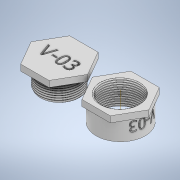
# Autodesk Inventor part: boltAndNut1_625x12-V03
Saved by Autodesk Inventor 2021.1 (Build 251245000, 245)
## iProperties
Created: 2020-08-22
Part Number: boltAndNut1_625x12-V03
Material: Generic
Document SubType Name: Modeling
Designer: robst
Density: 1 g/cm^3
Appearance: Default
Author: robst
Autodesk Inventor part; units mm, degrees
ref_plane "XZ Plane" through (0, 0, 0) normal (0, 1, 0) x (-1, 0, 0)
ref_plane "XY Plane" through (0, 0, 0) normal (0, 0, 1) x (1, 0, 0)
sketch "Sketch4" plane through (0, 0, 0) normal (0, 1, 0) x (-1, 0, 0)
  circle A0 centre (0, 0) radius 25.4
  circle A1 centre (0, 0) radius 19.7206
  dimension "d4" = 50.8
  dimension "d5" = 39.4411
  constraints: 2 centre point, 2 coincident
  measures "d4" diameter of A0
  measures "d5" diameter of A1
extrude "NutShaft" add sketch "Sketch4" against normal blind 25.4
sketch "Sketch6" plane through (0, 0, 0) normal (0, 0, 1) x (1, 0, 0)
  line L0 (19.7206, -25.4) -> (19.7206, 0) projected
  line L1 (19.7206, 2.1167) -> (20.8305, 2.7575)
  line L2 (20.8305, 2.9555) -> (19.7206, 3.5963)
  line L3 (19.7206, 3.5963) -> (19.7206, 2.1167)
  line L4 (0, -31.1993) -> (0, 9.3956) projected
  arc A0 (20.8305, 2.7575) -> (20.8305, 2.9555) centre (20.7734, 2.8565) ccw
  point P0 (0, 0)
  dimension "d33" = 60
  dimension "d35" = 0.1143
  dimension "d36" = 20.8877
  dimension "d37" = 2.1167
  dimension "d78" = 19.7206
  constraints: 6 end point, 2 point on circle, 2 tangent, 1 centre point, 1 collinear, 1 equal length, 1 vertical
  measures "d33" angle of L1 L2
  measures "d35" radius of A0
  measures "d37" distance of L1.start L0.end
  measures "d78" distance between parallel lines of L3 L4
coil "CoilForNut" sketch "Sketch6" operation cut axis through (0, -10, 0) along (0, -1, 0) pitch 2.1167 turns 14 hand right
sketch "Sketch7" plane through (0, 0, 0) normal (0, 1, 0) x (-1, 0, 0)
  line L0 (0, 0) -> (63.5, 0) construction
  line L1 (34.1706, 0) -> (48.8353, 25.4)
  line L2 (48.8353, 25.4) -> (78.1647, 25.4)
  line L3 (78.1647, 25.4) -> (92.8294, 0)
  line L4 (92.8294, 0) -> (78.1647, -25.4)
  line L5 (78.1647, -25.4) -> (48.8353, -25.4)
  line L6 (48.8353, -25.4) -> (34.1706, 0)
  dimension "d46" = 63.5
  dimension "d50" = 50.8
  constraints: 14 end point, 2 horizontal, 1 coincident, 13 other
  measures "d46" distance of L0.start L0.end
  measures "d50" distance between parallel lines of L2 L5
extrude "BoltHexHead" add sketch "Sketch7" against normal blind 6.35
sketch "Sketch8" plane through (0, -6.35, 0) normal (0, -1, 0) x (1, 0, 0)
  line L0 (-48.8353, 25.4) -> (-78.1647, 25.4) projected
  line L1 (-34.1706, 0) -> (-48.8353, 25.4) projected
  line L2 (-48.8353, -25.4) -> (-34.1706, 0) projected
  line L3 (-78.1647, -25.4) -> (-48.8353, -25.4) projected
  line L4 (-92.8294, 0) -> (-78.1647, -25.4) projected
  line L5 (-78.1647, 25.4) -> (-92.8294, 0) projected
  line L6 (-78.1647, 25.4) -> (-69.0759, -25.4) construction
  line L7 (-48.8353, 25.4) -> (-78.1647, -25.4) construction
  circle A0 centre (-63.5, 0) radius 20.4699
  point P0 (0, 0)
  dimension "d49" = 40.9397
  constraints: 4 end point, 1 centre point, 1 midpoint, 1 parallel, 1 point on line
  measures "d49" diameter of A0
extrude "BoltShaft" add sketch "Sketch8" along normal blind 19.05 contours A0
sketch "Sketch9" plane through (0, 0, 0) normal (0, 0, 1) x (1, 0, 0)
  line L0 (-43.0301, -6.35) -> (-43.0301, -25.4) projected
  line L1 (-83.9699, -25.4) -> (-43.0301, -25.4) projected
  line L2 (-43.0301, -27.5167) -> (-44.3116, -28.2565)
  line L3 (-44.3116, -28.5821) -> (-43.0301, -29.3219)
  line L4 (-43.0301, -29.3219) -> (-43.0301, -27.5167)
  line L5 (-63.5, -25.4) -> (-63.5, 0) construction
  line L6 (-78.1647, 0) -> (-48.8353, 0) construction
  arc A0 (-44.3116, -28.2565) -> (-44.3116, -28.5821) centre (-44.2176, -28.4193) ccw
  point P0 (0, 0)
  dimension "d53" = 60
  dimension "d54" = 0.188
  dimension "d56" = 20.4699
  dimension "d57" = 19.0944
  dimension "d66" = 2.1167
  constraints: 8 end point, 2 midpoint, 2 point on circle, 2 tangent, 1 centre point, 1 equal length
  measures "d53" angle of L2 L3
  measures "d54" radius of A0
  measures "d56" distance between parallel lines of L4 L5
  measures "d57" distance edge to line of A0 L5
  measures "d66" distance of L2.start L0.end
coil "CoilForBolt" sketch "Sketch9" operation cut axis through (-63.5, -25.4, 0) along (0, 1, 0) pitch 2.1167 turns 10 hand right
sketch "Sketch11" plane through (0, 0, 0) normal (0, 1, 0) x (1, 0, 0)
  line L0 (-78.1647, -25.4) -> (-92.8294, 0) construction
  line L1 (-48.8353, 25.4) -> (-34.1706, 0) construction
  line L2 (-92.8294, 0) -> (-34.1706, 0) construction
  line L3 (-70.9152, 6.35) -> (-75.2892, -6.35)
  line L4 (-75.2892, -6.35) -> (-77.1108, -6.35)
  line L5 (-77.1108, -6.35) -> (-81.4848, 6.35)
  line L6 (-81.4848, 6.35) -> (-79.6735, 6.35)
  line L7 (-79.6735, 6.35) -> (-76.1537, -4.199)
  line L8 (-76.1537, -4.199) -> (-72.6339, 6.35)
  line L9 (-72.6339, 6.35) -> (-70.9152, 6.35)
  line L10 (-65.265, -1.5643) -> (-70.0713, -1.5643)
  line L11 (-70.0713, -1.5643) -> (-70.0713, -0.0206)
  line L12 (-70.0713, -0.0206) -> (-65.265, -0.0206)
  line L13 (-65.265, -0.0206) -> (-65.265, -1.5643)
  spline S0 degree 2 poles (-55.6731, 0) (-55.6731, -3.4169) (-57.6594, -6.6176) (-59.7281, -6.6176) knots 0 0 0 1 2 2 2
  spline S1 degree 2 poles (-59.7281, -6.6176) (-61.8276, -6.6176) (-63.7933, -3.3551) (-63.7933, -0.0103) knots 0 0 0 1 2 2 2
  spline S2 degree 2 poles (-63.7933, -0.0103) (-63.7933, 3.4271) (-61.807, 6.6073) (-59.7281, 6.6073) knots 0 0 0 1 2 2 2
  spline S3 degree 2 poles (-59.7281, 6.6073) (-57.6389, 6.6073) (-55.6731, 3.3139) (-55.6731, 0) knots 0 0 0 1 2 2 2
  spline S4 degree 2 poles (-57.855, -3.8697) (-57.608, -3.2419) (-57.4021, -1.3071) (-57.4021, 0) knots 0 0 0 1 2 2 2
  spline S5 degree 2 poles (-57.4021, 0) (-57.4021, 1.3071) (-57.608, 3.2316) (-57.8653, 3.88) knots 0 0 0 1 2 2 2
  spline S6 degree 2 poles (-57.8653, 3.88) (-58.1226, 4.5284) (-59.0179, 5.1973) (-59.7281, 5.1973) knots 0 0 0 1 2 2 2
  spline S7 degree 2 poles (-59.7281, 5.1973) (-60.4382, 5.1973) (-61.3542, 4.5284) (-61.6218, 3.8594) knots 0 0 0 1 2 2 2
  spline S8 degree 2 poles (-61.6218, 3.8594) (-61.8791, 3.211) (-62.0643, 1.235) (-62.0643, -0.0103) knots 0 0 0 1 2 2 2
  spline S9 degree 2 poles (-62.0643, -0.0103) (-62.0643, -1.3482) (-61.8996, -3.139) (-61.632, -3.8388) knots 0 0 0 1 2 2 2
  spline S10 degree 2 poles (-61.632, -3.8388) (-61.385, -4.4975) (-60.4691, -5.2076) (-59.7281, -5.2076) knots 0 0 0 1 2 2 2
  spline S11 degree 2 poles (-59.7281, -5.2076) (-59.0282, -5.2076) (-58.1123, -4.5387) (-57.855, -3.8697) knots 0 0 0 1 2 2 2
  spline S12 degree 2 poles (-50.6199, 5.1459) (-51.083, 5.1459) (-51.999, 4.9194) (-52.4415, 4.7445) knots 0 0 0 1 2 2 2
  spline S13 degree 2 poles (-52.4415, 4.7445) (-52.8532, 4.5695) (-53.4604, 4.199) (-53.6971, 4.0344) knots 0 0 0 1 2 2 2
  line L14 (-53.6971, 4.0344) -> (-53.8, 4.0344)
  line L15 (-53.8, 4.0344) -> (-53.8, 5.8354)
  spline S14 degree 2 poles (-53.8, 5.8354) (-53.2443, 6.1339) (-51.3403, 6.6176) (-50.4861, 6.6176) knots 0 0 0 1 2 2 2
  spline S15 degree 2 poles (-50.4861, 6.6176) (-49.6216, 6.6176) (-48.3351, 6.2677) (-47.8103, 5.8972) knots 0 0 0 1 2 2 2
  spline S16 degree 2 poles (-47.8103, 5.8972) (-47.2545, 5.4958) (-46.6782, 4.3328) (-46.6782, 3.5506) knots 0 0 0 1 2 2 2
  spline S17 degree 2 poles (-46.6782, 3.5506) (-46.6782, 2.5009) (-48.0573, 0.916) (-49.0247, 0.7101) knots 0 0 0 1 2 2 2
  line L16 (-49.0247, 0.7101) -> (-49.0247, 0.5866)
  spline S18 degree 2 poles (-49.0247, 0.5866) (-48.6233, 0.5043) (-47.7073, 0.1338) (-47.3162, -0.2367) knots 0 0 0 1 2 2 2
  spline S19 degree 2 poles (-47.3162, -0.2367) (-46.9252, -0.5969) (-46.4312, -1.7496) (-46.4312, -2.5832) knots 0 0 0 1 2 2 2
  spline S20 degree 2 poles (-46.4312, -2.5832) (-46.4312, -3.4374) (-47.0178, -4.8886) (-47.553, -5.4443) knots 0 0 0 1 2 2 2
  spline S21 degree 2 poles (-47.553, -5.4443) (-48.1087, -6.0207) (-49.6833, -6.6176) (-50.6816, -6.6176) knots 0 0 0 1 2 2 2
  spline S22 degree 2 poles (-50.6816, -6.6176) (-51.6388, -6.6176) (-53.5119, -6.1545) (-54.15, -5.8354) knots 0 0 0 1 2 2 2
  line L17 (-54.15, -5.8354) -> (-54.15, -4.0344)
  line L18 (-54.15, -4.0344) -> (-54.0265, -4.0344)
  spline S23 degree 2 poles (-54.0265, -4.0344) (-53.4913, -4.4254) (-51.6799, -5.1459) (-50.7846, -5.1459) knots 0 0 0 1 2 2 2
  spline S24 degree 2 poles (-50.7846, -5.1459) (-50.2597, -5.1459) (-49.2099, -4.8165) (-48.86, -4.4357) knots 0 0 0 1 2 2 2
  spline S25 degree 2 poles (-48.86, -4.4357) (-48.5204, -4.0549) (-48.1602, -3.1493) (-48.1602, -2.4597) knots 0 0 0 1 2 2 2
  spline S26 degree 2 poles (-48.1602, -2.4597) (-48.1602, -1.7702) (-48.5615, -0.8748) (-48.9218, -0.6175) knots 0 0 0 1 2 2 2
  spline S27 degree 2 poles (-48.9218, -0.6175) (-49.282, -0.3602) (-50.2597, -0.1647) (-50.836, -0.1647) knots 0 0 0 1 2 2 2
  line L19 (-50.836, -0.1647) -> (-51.5564, -0.1647)
  line L20 (-51.5564, -0.1647) -> (-51.5564, 1.2453)
  line L21 (-51.5564, 1.2453) -> (-50.9904, 1.2453)
  spline S28 degree 2 poles (-50.9904, 1.2453) (-49.848, 1.2453) (-48.4072, 2.3362) (-48.4072, 3.3757) knots 0 0 0 1 2 2 2
  spline S29 degree 2 poles (-48.4072, 3.3757) (-48.4072, 3.8594) (-48.7777, 4.5489) (-49.0761, 4.7548) knots 0 0 0 1 2 2 2
  spline S30 degree 2 poles (-49.0761, 4.7548) (-49.3952, 4.9709) (-50.1774, 5.1459) (-50.6199, 5.1459) knots 0 0 0 1 2 2 2
  point P0 (0, 0)
  constraints: 2 end point, 2 horizontal
extrude "EmbossForBolt" cut sketch "Sketch11" against normal blind 2.54
ref_plane "Work Plane4" through (25.4, 0, 0) normal (1, 0, 0) x (0, 1, 0)
sketch "Sketch12" plane through (25.4, 0, 0) normal (1, 0, 0) x (0, 1, 0)
  line L0 (0, 25.4) -> (-25.4, 25.4)
  line L1 (0, -25.4) -> (0, 25.4)
  line L2 (0, -25.4) -> (-25.4, -25.4)
  line L3 (-25.4, 25.4) -> (-25.4, -25.4) projected
  line L4 (-12.7, 25.4) -> (-12.7, -25.4) construction
  line L5 (-17.78, -5.9322) -> (-7.62, -9.4313)
  line L6 (-7.62, -9.4313) -> (-7.62, -10.8887)
  line L7 (-7.62, -10.8887) -> (-17.78, -14.3878)
  line L8 (-17.78, -14.3878) -> (-17.78, -12.9388)
  line L9 (-17.78, -12.9388) -> (-9.3408, -10.1229)
  line L10 (-9.3408, -10.1229) -> (-17.78, -7.3071)
  line L11 (-17.78, -7.3071) -> (-17.78, -5.9322)
  line L12 (-11.4485, -1.412) -> (-11.4485, -5.257)
  line L13 (-11.4485, -5.257) -> (-12.6835, -5.257)
  line L14 (-12.6835, -5.257) -> (-12.6835, -1.412)
  line L15 (-12.6835, -1.412) -> (-11.4485, -1.412)
  spline S0 degree 2 poles (-12.7, 6.2615) (-9.9665, 6.2615) (-7.4059, 4.6724) (-7.4059, 3.0175) knots 0 0 0 1 2 2 2
  spline S1 degree 2 poles (-7.4059, 3.0175) (-7.4059, 1.3379) (-10.0159, -0.2347) (-12.6918, -0.2347) knots 0 0 0 1 2 2 2
  spline S2 degree 2 poles (-12.6918, -0.2347) (-15.4417, -0.2347) (-17.9858, 1.3544) (-17.9858, 3.0175) knots 0 0 0 1 2 2 2
  spline S3 degree 2 poles (-17.9858, 3.0175) (-17.9858, 4.6889) (-15.3512, 6.2615) (-12.7, 6.2615) knots 0 0 0 1 2 2 2
  spline S4 degree 2 poles (-9.6042, 4.516) (-10.1065, 4.7136) (-11.6544, 4.8783) (-12.7, 4.8783) knots 0 0 0 1 2 2 2
  spline S5 degree 2 poles (-12.7, 4.8783) (-13.7456, 4.8783) (-15.2853, 4.7136) (-15.804, 4.5078) knots 0 0 0 1 2 2 2
  spline S6 degree 2 poles (-15.804, 4.5078) (-16.3227, 4.3019) (-16.8579, 3.5856) (-16.8579, 3.0175) knots 0 0 0 1 2 2 2
  spline S7 degree 2 poles (-16.8579, 3.0175) (-16.8579, 2.4494) (-16.3227, 1.7167) (-15.7875, 1.5026) knots 0 0 0 1 2 2 2
  spline S8 degree 2 poles (-15.7875, 1.5026) (-15.2688, 1.2968) (-13.688, 1.1486) (-12.6918, 1.1486) knots 0 0 0 1 2 2 2
  spline S9 degree 2 poles (-12.6918, 1.1486) (-11.6214, 1.1486) (-10.1888, 1.2803) (-9.6289, 1.4944) knots 0 0 0 1 2 2 2
  spline S10 degree 2 poles (-9.6289, 1.4944) (-9.102, 1.692) (-8.5339, 2.4247) (-8.5339, 3.0175) knots 0 0 0 1 2 2 2
  spline S11 degree 2 poles (-8.5339, 3.0175) (-8.5339, 3.5774) (-9.0691, 4.3102) (-9.6042, 4.516) knots 0 0 0 1 2 2 2
  spline S12 degree 2 poles (-16.8167, 10.3041) (-16.8167, 9.9336) (-16.6356, 9.2008) (-16.4956, 8.8468) knots 0 0 0 1 2 2 2
  spline S13 degree 2 poles (-16.4956, 8.8468) (-16.3556, 8.5174) (-16.0592, 8.0317) (-15.9275, 7.8423) knots 0 0 0 1 2 2 2
  line L16 (-15.9275, 7.8423) -> (-15.9275, 7.76)
  line L17 (-15.9275, 7.76) -> (-17.3683, 7.76)
  spline S14 degree 2 poles (-17.3683, 7.76) (-17.6071, 8.2046) (-17.9941, 9.7277) (-17.9941, 10.4111) knots 0 0 0 1 2 2 2
  spline S15 degree 2 poles (-17.9941, 10.4111) (-17.9941, 11.1027) (-17.7141, 12.1319) (-17.4177, 12.5518) knots 0 0 0 1 2 2 2
  spline S16 degree 2 poles (-17.4177, 12.5518) (-17.0966, 12.9964) (-16.1663, 13.4575) (-15.5405, 13.4575) knots 0 0 0 1 2 2 2
  spline S17 degree 2 poles (-15.5405, 13.4575) (-14.7007, 13.4575) (-13.4328, 12.3542) (-13.2681, 11.5803) knots 0 0 0 1 2 2 2
  line L18 (-13.2681, 11.5803) -> (-13.1693, 11.5803)
  spline S18 degree 2 poles (-13.1693, 11.5803) (-13.1034, 11.9014) (-12.807, 12.6341) (-12.5106, 12.947) knots 0 0 0 1 2 2 2
  spline S19 degree 2 poles (-12.5106, 12.947) (-12.2225, 13.2599) (-11.3003, 13.6551) (-10.6334, 13.6551) knots 0 0 0 1 2 2 2
  spline S20 degree 2 poles (-10.6334, 13.6551) (-9.95, 13.6551) (-8.7891, 13.1858) (-8.3445, 12.7576) knots 0 0 0 1 2 2 2
  spline S21 degree 2 poles (-8.3445, 12.7576) (-7.8835, 12.313) (-7.4059, 11.0533) (-7.4059, 10.2547) knots 0 0 0 1 2 2 2
  spline S22 degree 2 poles (-7.4059, 10.2547) (-7.4059, 9.489) (-7.7764, 7.9905) (-8.0317, 7.48) knots 0 0 0 1 2 2 2
  line L19 (-8.0317, 7.48) -> (-9.4725, 7.48)
  line L20 (-9.4725, 7.48) -> (-9.4725, 7.5788)
  spline S23 degree 2 poles (-9.4725, 7.5788) (-9.1596, 8.007) (-8.5833, 9.456) (-8.5833, 10.1724) knots 0 0 0 1 2 2 2
  spline S24 degree 2 poles (-8.5833, 10.1724) (-8.5833, 10.5923) (-8.8468, 11.4321) (-9.1514, 11.712) knots 0 0 0 1 2 2 2
  spline S25 degree 2 poles (-9.1514, 11.712) (-9.456, 11.9837) (-10.1806, 12.2719) (-10.7322, 12.2719) knots 0 0 0 1 2 2 2
  spline S26 degree 2 poles (-10.7322, 12.2719) (-11.2839, 12.2719) (-12.0002, 11.9508) (-12.206, 11.6626) knots 0 0 0 1 2 2 2
  spline S27 degree 2 poles (-12.206, 11.6626) (-12.4118, 11.3744) (-12.5683, 10.5923) (-12.5683, 10.1312) knots 0 0 0 1 2 2 2
  line L21 (-12.5683, 10.1312) -> (-12.5683, 9.5548)
  line L22 (-12.5683, 9.5548) -> (-13.6962, 9.5548)
  line L23 (-13.6962, 9.5548) -> (-13.6962, 10.0077)
  spline S28 degree 2 poles (-13.6962, 10.0077) (-13.6962, 10.9216) (-14.569, 12.0743) (-15.4006, 12.0743) knots 0 0 0 1 2 2 2
  spline S29 degree 2 poles (-15.4006, 12.0743) (-15.7875, 12.0743) (-16.3392, 11.7779) (-16.5038, 11.5391) knots 0 0 0 1 2 2 2
  spline S30 degree 2 poles (-16.5038, 11.5391) (-16.6767, 11.2839) (-16.8167, 10.6581) (-16.8167, 10.3041) knots 0 0 0 1 2 2 2
  point P0 (0, 0)
  constraints: 8 end point, 2 midpoint, 1 coincident, 1 vertical
emboss "EmbossForNut" sketch "Sketch12" operation cut depth 2.54 direction (-1, 0, 0) wrap yes faces at (-25.3176, -16.9333, -2.0439) contours L5 L6 L7 L8 L9 L10 L11 | L12 L13 L14 L15 | S0 S1 S2 S3 | S12 S13 L16 L17 S14 S15 S16 S17 L18 S18 S19 S20 S21 S22 L19 L20 S23 S24 S25 S26 S27 L21 L22 L23 S28 S29 S30
sketch "Sketch13" plane through (0, 0, 0) normal (0, 1, 0) x (1, 0, 0)
  line L0 (29.3294, 0) -> (14.6647, -25.4)
  line L1 (14.6647, -25.4) -> (-14.6647, -25.4)
  line L2 (-14.6647, -25.4) -> (-29.3294, 0)
  line L3 (-29.3294, 0) -> (-14.6647, 25.4)
  line L4 (-14.6647, 25.4) -> (14.6647, 25.4)
  line L5 (14.6647, 25.4) -> (29.3294, 0)
  line L6 (19.9576, 11.1478) -> (22.1751, 12.3864) projected
  circle A0 centre (0, 0) radius 22.86
  dimension "d73" = 50.8
  constraints: 12 end point, 2 coincident, 1 horizontal, 16 other
  measures "d73" distance between parallel lines of L1 L4
extrude "NutHexHead" add sketch "Sketch13" against normal blind 6.35
sketch "Sketch14" plane through (0, -25.4, 0) normal (0, -1, 0) x (1, 0, 0)
  line L0 (-34.1706, 0) -> (-48.8353, 25.4) projected
  line L1 (-48.8353, -25.4) -> (-34.1706, 0) projected
  line L2 (-78.1647, -25.4) -> (-48.8353, -25.4) projected
  line L3 (-92.8294, 0) -> (-78.1647, -25.4) projected
  line L4 (-78.1647, 25.4) -> (-92.8294, 0) projected
  line L5 (-48.8353, 25.4) -> (-78.1647, 25.4) projected
  line L6 (-48.8353, 25.4) -> (-78.1647, -25.4) construction
  line L7 (-92.8294, 0) -> (-78.1647, 25.4) construction
  line L8 (-48.8353, -25.4) -> (-78.1647, 25.4) construction
  circle A0 centre (-63.5, 0) radius 12.7
  point P0 (0, 0)
  constraints: 4 end point, 1 centre point, 1 midpoint
extrude "HoleForBolt" cut sketch "Sketch14" against normal blind 19.05 contours A0
equation "\"d4\" = nutOutsideDiameter"
equation "\"d5\" = b2MinorDiameterMax"
equation "\"d35\" = b2RootRadiusAvg"
equation "\"d36\" = 0.5 * b2MajorDiameterMax"
equation "\"d37\" = pitch"
equation "\"d38\" = pitch"
equation "\"d39\" = cuttingLengthOfNut"
equation "\"d46\" = distanceBetweenCenters"
equation "\"d50\" = hexNutSize"
equation "\"d49\" = a2MajorDiameterMin"
equation "\"d54\" = a2RootRadiusAvg"
equation "\"d56\" = 0.5 * a2MajorDiameterMin"
equation "\"d57\" = 0.5 * a2MinorDiameterMin"
equation "\"d66\" = pitch"
equation "\"d58\" = pitch"
equation "\"b2ThreadDepthMin\" = 0.91694"
equation "\"d73\" = hexNutSize"
equation "\"d74\" = hexNutHeight"
equation "\"a2MajorDiameterMax\" = 41.22928"
equation "\"a2MajorDiameterMin\" = 40.93972"
equation "\"a2PitchDiameterMax\" = 39.85514"
equation "\"a2PitchDiamterMin\" = 39.70528"
equation "\"a2MinorDiameterMax\" = 38.7096"
equation "\"a2MinorDiameterMin\" = 38.1889"
equation "\"a2CrestFlatMax\" = 0.4318"
equation "\"a2CrestFlatMin\" = 0.1778"
equation "\"a2RootFlatMax\" = 0.38862"
equation "\"a2RootFlatMin\" = 0.26416"
equation "\"a2RootRadiusMax\" = 0.22352"
equation "\"a2RootRadiusMin\" = 0.1524"
equation "\"a2ThreadDepthMax\" = 1.52146"
equation "\"a2ThreadDepthMin\" = 1.11506"
equation "\"b2MajorDiameterMax\" = 41.77538"
equation "\"b2MajorDiameterMin\" = 41.275"
equation "\"b2PitchDiameterMax\" = 40.09644"
equation "\"b2PitchDiameterMin\" = 39.90086"
equation "\"b2MinorDiameterMax\" = 39.44112"
equation "\"b2MinorDiameterMin\" = 38.98392"
equation "\"b2CrestFlatMax\" = 7.9502"
equation "\"b2CrestFlatMin\" = 0.41656"
equation "\"b2RootFlatMax\" = 0.26416"
equation "\"b2RootFlatMin\" = 0.0889"
equation "\"b2RootRadiusMax\" = 0.1524"
equation "\"b2RootRadiusMin\" = 0.0762"
equation "\"b2ThreadDepthMax\" = 1.397"
equation "\"b2MajorDiameter\" = 0.5 * b2MajorDiameterMin + 0.5 * b2MajorDiameterMax"
equation "\"b2MinorDiameter\" = 0.5 * b2MinorDiameterMin + 0.5 * b2MinorDiameterMax"
equation "\"b2RootRadiusAvg\" = 0.5 * b2RootRadiusMin + 0.5 * b2RootRadiusMax"
equation "\"a2MajorDiameter\" = 0.5 * a2MajorDiameterMin + 0.5 * a2MajorDiameterMax"
equation "\"a2MinorDiameter\" = 0.5 * a2MinorDiameterMin + 0.5 * a2MinorDiameterMax"
equation "\"a2RootRadiusAvg\" = 0.5 * a2RootRadiusMin + 0.5 * a2RootRadiusMax"
equation "\"nutOutsideDiameter\" = 50.8"
equation "\"d70\" = 0.5 * nutOutsideDiameter"
equation "\"heightOfNut\" = 25.4"
equation "\"hexNutSize\" = 50.8"
equation "\"hexNutHeight\" = 6.35"
equation "\"distanceBetweenCenters\" = 63.5"
equation "\"pitch\" = 2.116667"
equation "\"cuttingLengthOfNut\" = 29.633333"
body "Solid2"
